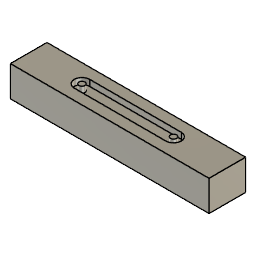
hexbug_3.5cm_mold v1 (Autodesk Fusion 360 design; units mm, degrees)
Autodesk Fusion 360 part; units mm, degrees
note: some values were not read from the file. Set by a fixed rule: which sketch regions a step uses.
sketch "Sketch1" plane through (0, 0, 0) normal (0, 0, 1) x (1, 0, 0)
  line L0 (0, 0) -> (-65, 0)
  line L1 (-65, 0) -> (-65, 12)
  line L2 (-65, 12) -> (0, 12)
  line L3 (0, 12) -> (0, 0)
  dimension "d1" = 12
  dimension "d2" = 65
  constraint horizontal L0
  constraint vertical L1
  constraint horizontal L2
  constraint vertical L3
  constraint coincident L0.start L3.end
  measures "d1" distance of L0.start L2.end
  measures "d2" distance of L1.end L2.end
extrude "Extrude1" add sketch "Sketch1" along normal blind 10
sketch "Sketch2" plane through (0, 0, 10) normal (0, 0, 1) x (-1, 0, 0)
  line L0 (0, -12) -> (65, -12)
  line L1 (65, -12) -> (65, 0)
  line L2 (65, 0) -> (0, 0)
  line L3 (0, 0) -> (0, -12)
  line L4 (0, -6) -> (65, -6)
  line L5 (32.5, 0) -> (32.5, -12)
  line L6 (32.5, -6) -> (32.5, -8.5)
  line L7 (32.5, -6) -> (32.5, -3.5)
  line L8 (32.5, -8.5) -> (47.5, -8.5)
  line L9 (32.5, -3.5) -> (47.5, -3.5)
  line L10 (32.5, -3.5) -> (17.5, -3.5)
  line L11 (32.5, -8.5) -> (17.5, -8.5)
  circle A0 centre (17.5972, -6) radius 2.5019
  circle A1 centre (47.5665, -6) radius 2.5009
  circle A2 centre (17.5972, -6) radius 1
  circle A3 centre (47.5665, -6) radius 1
  dimension "d5" = 2.5
  dimension "d6" = 2.5
  dimension "d7" = 15
  dimension "d8" = 15
  dimension "d9" = 15
  dimension "d10" = 15
  dimension "d11" = 2
  dimension "d12" = 2
  constraint midpoint L3 L4.start
  constraint midpoint L1 L4.end
  constraint midpoint L2 L5.start
  constraint midpoint L0 L5.end
  constraint midpoint L4 L6.start
  constraint coincident L5 L6.end
  constraint perpendicular L4 L7
  constraint perpendicular L5 L8
  constraint perpendicular L5 L9
  constraint perpendicular L5 L10
  constraint perpendicular L6 L11
  constraint coincident L4 A0.centre
  constraint coincident L11.end A0
  constraint coincident L4 A1.centre
  constraint coincident L8.end A1
  constraint concentric A0 A2
  constraint concentric A1 A3
  measures "d5" distance of L6.start L6.end
  measures "d6" distance of L6.start L7.end
  measures "d7" distance of L6.end L8.end
  measures "d8" distance of L7.end L9.end
  measures "d9" distance of L7.end L10.end
  measures "d10" distance of L6.end L11.end
  measures "d11" diameter of A2
  measures "d12" diameter of A3
extrude "Extrude2" cut sketch "Sketch2" against normal blind 2 contours L4 A0 A2 | L4 L5 L7 L10 A0 | L4 L5 L6 L11 A0 | L4 L5 L6 L8 A1 | L4 A0 A2 | L4 L5 L7 L9 A1 | L4 A1 A3 | L4 A1 A3
